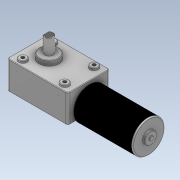
# Autodesk Inventor part: SteeringMotor
Saved by Autodesk Inventor 2020 (Build 240168000, 168)
## iProperties
Created: 2019-12-15
Part Number: SteeringMotor
Material: Generic
Document SubType Name: Modeling
Designer: Kjell
Density: 3.21833 g/cm^3
Appearance: Aluminum Cast
Mass: 350 g
Surface Area: 174.384 cm^2
Volume: 108.752 cm^3
Author: Kjell
Autodesk Inventor part; units mm, degrees
ref_plane "YZ Plane" through (0, 0, 0) normal (1, 0, 0) x (0, 1, 0)
ref_plane "XZ Plane" through (0, 0, 0) normal (0, 1, 0) x (-1, 0, 0)
ref_plane "XY Plane" through (0, 0, 0) normal (0, 0, 1) x (1, 0, 0)
sketch "Sketch1" plane through (0, 0, 0) normal (0, 0, 1) x (1, 0, 0)
  line L0 (-20, 20) -> (38, 20)
  line L1 (38, 20) -> (38, -20)
  line L2 (38, -20) -> (-20, -20)
  line L3 (-20, -20) -> (-20, 20)
  line L4 (-20, 20) -> (38, -20) construction
  line L5 (38, 20) -> (-20, -20) construction
  point P0 (0, 0)
  point P1 (9, 0)
  point P2 (9, 0)
  dimension "GearboxLength" = 58
  dimension "Gearbox_Width" = 40
  dimension "AxelOffset" = 20
  constraints: 12 end point, 3 midpoint, 2 parallel, 1 horizontal, 1 horizontal alignment, 1 perpendicular
  measures "GearboxLength" distance of L1.end L2.end
  measures "Gearbox_Width" distance of L0.end L1.end
  measures "AxelOffset" distance from line of point (0, 0) L3
extrude "GearboxBody" add sketch "Sketch1" along normal mid plane 26.8
sketch "Sketch2" plane through (0, 0, 13.4) normal (0, 0, 1) x (1, 0, 0)
  line L0 (-20, -20) -> (38, -20) projected
  line L1 (-20, 20) -> (-20, -20) projected
  circle A0 centre (-11, -14) radius 4
  circle A1 centre (29, -14) radius 4
  circle A2 centre (-11, 14) radius 4
  circle A3 centre (29, 14) radius 4
  line L2 (0, 0) -> (-32.2431, 0) construction
  dimension "d5" = 8
  dimension "d6" = 11
  dimension "d9" = 40
  dimension "d12" = 28
  constraints: 4 centre point, 2 end point, 2 horizontal, 1 vertical, 7 other
  measures "d5" diameter of A0
  measures "d6" horizontal distance of A0.centre L2.start
  measures "d9" distance of A0.centre A1.centre
  measures "d12" distance of A0.centre A2.centre
extrude "MountBosses" add sketch "Sketch2" along normal blind 2 draft -5
sketch "Sketch3" plane through (0, 0, 13.4) normal (0, 0, 1) x (1, 0, 0)
  circle A0 centre (0, 0) radius 9.4
  dimension "d17" = 18.8
  constraints: 1 centre point, 1 coincident
  measures "d17" diameter of A0
extrude "AxelBoss" add sketch "Sketch3" along normal blind 4.5 draft -5
sketch "Sketch4" plane through (0, 0, 17.9) normal (0, 0, 1) x (1, 0, 0)
  circle A0 centre (0, 0) radius 9.0063 projected
  circle A1 centre (0, 0) radius 4
  dimension "d20" = 8
  constraints: 1 centre point, 1 coincident
  measures "d20" diameter of A1
extrude "Axel" add sketch "Sketch4" along normal blind 15 contours A1
sketch "Sketch5" plane through (0, 0, 32.9) normal (0, 0, 1) x (1, 0, 0)
  circle A0 centre (0, 0) radius 4 projected
  line L0 (-3, -2.6458) -> (-3, 2.6458)
  line L1 (-3, -2.6458) -> (2.2915, -2.6458) construction
  line L2 (-3, 0) -> (4.7781, 0) construction
  point P0 (4, 0)
  dimension "d23" = 90
  dimension "d24" = 7
  constraints: 6 end point, 3 point on circle, 2 horizontal, 1 midpoint, 1 perpendicular, 1 point on line
  measures "d23" angle of L1 L0
  measures "d24" distance from line of L0 A0.end
extrude "AxelFlat" cut sketch "Sketch5" against normal blind 13 contours L0 A0 picked at (-3.1815, -0.6179)
sketch "Sketch6" plane through (-11, -14, 15.4) normal (0, 0, 1) x (1, 0, 0)
  circle A0 centre (0, 0) radius 3.825 construction
  circle A1 centre (40, 0) radius 3.825 construction
  circle A2 centre (40, 28) radius 3.825 construction
  circle A3 centre (0, 28) radius 3.825 construction
  point P0 (11, 14)
  constraints: 4 coincident
hole "MountHoles" at (-11, -14, 15.4) at (29, -14, 15.4) at (29, 14, 15.4) at (-11, 14, 15.4) direction (0, 0, -1) diameter 3.242 depth 8 thread size "M4x0.7" class "6H" standard "ISO Metric profile"
fillet "BossFillets" radius 0.5 5 edges at (-14.825, -14, 15.4) (25.175, -14, 15.4) (25.175, 14, 15.4) (-14.825, 14, 15.4) (-9.0063, 0, 17.9)
chamfer "AxelChamfer" distance 0.5 angle 45 3 edges at (1.4142, -3.7417, 32.9) (1.4142, 3.7417, 32.9) (-3, 0, 32.9)
mirror "Mirror1" about plane through (0, 0, 0) normal (0, 0, 1) of "MountBosses", "MountHoles", "AxelBoss", "BossFillets"
fillet "Fillet1" radius 2 4 edges at (38, -20, 0) (-20, -20, 0) (38, 20, 0) (-20, 20, 0)
fillet "Fillet1" radius 0.5 8 edges at (9, -20, 13.4) (38, 0, 13.4) (9, 20, 13.4) (-20, 0, 13.4) (9, -20, -13.4) (-20, 0, -13.4) (9, 20, -13.4) (38, 0, -13.4)
sketch "Sketch7" plane through (38, -20, 13.4) normal (1, 0, 0) x (0, 0, -1)
  line L0 (0, 0) -> (0, 40) projected
  circle A0 centre (17.5, 20) radius 15.5
  point P0 (13.4, 20)
  dimension "MotorDia" = 31
  dimension "d35" = 17.5
  constraints: 1 centre point, 1 horizontal alignment
  measures "MotorDia" diameter of A0
  measures "d35" distance from line of L0 A0.centre
extrude "MotorBody" add sketch "Sketch7" along normal blind 57.2 separate body
sketch "Sketch8" plane through (95.2, 0, -4.1) normal (1, 0, 0) x (0, 0, -1)
  circle A0 centre (0, 0) radius 15.5 projected
  circle A1 centre (0, 0) radius 6
  point P0 (-4.1, 0)
  dimension "d38" = 12
  constraints: 1 centre point, 1 coincident
  measures "d38" diameter of A1
extrude "Extrusion7" add sketch "Sketch8" along normal blind 2 draft -5 contours A1 bodies 2
sketch "Sketch9" plane through (97.2, 0, -4.1) normal (1, 0, 0) x (0, 0, -1)
  circle A0 centre (0, 0) radius 5.825 projected
  circle A1 centre (0, 0) radius 2
  point P0 (-4.1, 0)
  dimension "d41" = 4
  constraints: 1 centre point, 1 coincident
  measures "d41" diameter of A1
extrude "Extrusion8" add sketch "Sketch9" along normal blind 1 contours A1 bodies 2
fillet "Fillet3" radius 1 2 edges at (38, 0, 11.4) (95.2, 0, 11.4)
fillet "Fillet4" radius 0.5 2 edges at (97.2, 0, 1.725) (98.2, 0, -2.1)
combine bodies "Combine1" operation type add bodies to combine 1 2
sketch "Sketch10" plane through (29, -14, 7.4) normal (0, 0, 1) x (1, 0, 0)
  point P0 (0, 0)
sketch "Sketch11" plane through (29, 14, 7.4) normal (0, 0, 1) x (1, 0, 0)
  point P0 (0, 0)
sketch "Sketch12" plane through (-11, 14, 7.4) normal (0, 0, 1) x (1, 0, 0)
  point P0 (0, 0)
sketch "Sketch13" plane through (-11, -14, 7.4) normal (0, 0, 1) x (1, 0, 0)
  point P0 (0, 0)
body "Solid1"
